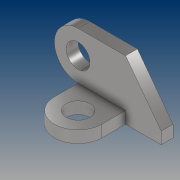
# Autodesk Inventor part: 25
Saved by Autodesk Inventor 2020.2 (Build 242310000, 310)
## iProperties
Created: 2020-09-17
Part Number: 25
Material: 鋼、碳鋼
Document SubType Name: Modeling
Designer: user
Density: 7.85 g/cm^3
Appearance: 半拋光
Mass: 339.773 g
Surface Area: 129.699 cm^2
Volume: 43.2832 cm^3
Author: user
Autodesk Inventor part; units mm, degrees
ref_plane "YZ Plane" through (0, 0, 0) normal (1, 0, 0) x (0, 1, 0)
ref_plane "XZ Plane" through (0, 0, 0) normal (0, 1, 0) x (-1, 0, 0)
ref_plane "XY Plane" through (0, 0, 0) normal (0, 0, 1) x (1, 0, 0)
sketch "草圖1" plane through (0, 0, 0) normal (0, 0, 1) x (1, 0, 0)
  circle A0 centre (0, 0) radius 20
  line L0 (0, -20) -> (0, -30)
  line L1 (0, -30) -> (70, -30)
  line L2 (70, -30) -> (70, -20)
  line L3 (70, -20) -> (40, 20)
  line L4 (40, 20) -> (0, 20)
  dimension "d0" = 40
  dimension "d1" = 10
  dimension "d2" = 70
  dimension "d3" = 40
  dimension "d4" = 10
  constraints: 10 end point, 2 perpendicular, 2 point on circle, 1 centre point, 1 coincident, 1 horizontal, 1 point on line, 1 vertical, 1 vertical alignment
  measures "d0" diameter of A0
  measures "d1" distance of L0.start L0.end
  measures "d2" horizontal distance of L2.end A0.centre
  measures "d3" distance of L3.end L4.end
  measures "d4" distance of L1.end L2.end
extrude "擠出1" add sketch "草圖1" along normal blind 10
sketch "草圖2" plane through (0, 0, 10) normal (0, 0, 1) x (1, 0, 0)
  arc A0 (0, 20) -> (0, -20) centre (0, 0) ccw projected
  constraints: 1 coincident
hole "孔1" at (0, 0, 10) direction (0, 0, -1) diameter 20 end through all
sketch "草圖3" plane through (0, -30, 0) normal (0, -1, 0) x (1, 0, 0)
  line L0 (70, 10) -> (70, 0) projected
  line L1 (70, 0) -> (0, 0) projected
  line L2 (0, 0) -> (0, 10) projected
  line L3 (0, 10) -> (70, 10) projected
  circle A0 centre (20, 30) radius 20
  line L4 (0, 30) -> (40, 30)
  line L5 (40, 30) -> (40, 0)
  line L6 (40, 0) -> (0, 0)
  line L7 (0, 0) -> (0, 30)
  line L8 (0, 0) -> (70, 0) projected
  line L9 (0, 0) -> (0, 10) projected
  point P0 (40, 10)
  point P1 (40, 30)
  dimension "d14" = 40
  dimension "d15" = 30
  constraints: 8 end point, 2 collinear, 2 parallel, 2 vertical, 1 horizontal, 1 perpendicular, 3 other
  measures "d15" distance between parallel lines of L4 L1
extrude "擠出2" add sketch "草圖3" against normal blind 10 contours L3 A0 L5 | L3 L7 A0 | A0 L4 | L4 A0
sketch "草圖4" plane through (0, -20, 0) normal (0, 1, 0) x (1, 0, 0)
  arc A0 (0, -30) -> (40, -30) centre (20, -30) ccw projected
  point P0 (0, 0)
  constraints: 1 coincident
hole "孔2" at (20, -20, 30) direction (0, -1, 0) diameter 20 end through all
